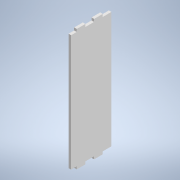
# Autodesk Inventor part: motorkap
Saved by Autodesk Inventor 2021 (Build 250183000, 183)
## iProperties
Created: 2022-02-02
Part Number: motorkap
Material: Generic
Document SubType Name: Modeling
Designer: ryan
Density: 1 g/cm^3
Appearance: Default
Author: ryan
Autodesk Inventor part; units mm, degrees
ref_plane "YZ Plane" through (0, 0, 0) normal (1, 0, 0) x (0, 1, 0)
ref_plane "XZ Plane" through (0, 0, 0) normal (0, 1, 0) x (-1, 0, 0)
ref_plane "XY Plane" through (0, 0, 0) normal (0, 0, 1) x (1, 0, 0)
sketch "Sketch1" plane through (0, 0, 0) normal (0, 1, 0) x (-1, 0, 0)
  line L0 (0, 0) -> (0, -10)
  line L1 (0, -10) -> (3, -10)
  line L2 (0, 0) -> (0, 10)
  line L3 (0, 10) -> (0, 20)
  line L4 (0, 20) -> (0, 30)
  line L5 (0, 30) -> (0, 36.5)
  line L6 (0, 36.5) -> (3, 36.5)
  line L7 (3, 36.5) -> (3, -10)
  line L8 (3, 30) -> (0, 30)
  line L9 (0, 20) -> (3, 20)
  line L10 (0, 10) -> (3, 10)
  line L11 (0, 0) -> (3, 0)
  dimension "d0" = 10
  dimension "d1" = 3
  dimension "d2" = 10
  dimension "d3" = 10
  dimension "d4" = 10
  dimension "d5" = 6.5
  dimension "d6" = 3
  constraints: 24 end point, 6 perpendicular, 6 point on line, 3 vertical
  measures "d0" distance of L0.start L0.end
  measures "d1" distance of L0.end L1.end
  measures "d2" distance of L0.start L2.end
  measures "d3" distance of L2.end L3.end
  measures "d4" distance of L3.end L4.end
  measures "d5" distance of L4.end L5.end
  measures "d6" distance of L5.end L6.end
extrude "Extrusion1" add sketch "Sketch1" along normal blind 3 contours L2 L10 L7 L11 | L4 L8 L7 L9
sketch "Sketch2" plane through (0, 3, 0) normal (0, 1, 0) x (1, 0, 0)
  line L0 (0, 0) -> (0, 10)
  line L1 (-3, -20) -> (-3, -30) projected
  line L2 (0, 10) -> (-3, 10)
  line L3 (-3, 10) -> (-3, -30)
  line L4 (-3, -30) -> (0, -30)
  line L5 (0, -30) -> (0, 10)
  line L6 (0, -30) -> (0, -36.5)
  line L7 (0, -36.5) -> (-3, -36.5)
  line L8 (-3, -36.5) -> (-3, -30)
  line L9 (-3, -30) -> (0, -30)
  line L10 (0, -30) -> (0, -36.5)
  dimension "d9" = 10
  dimension "d10" = 6.5
  constraints: 20 end point, 4 parallel, 2 horizontal, 2 perpendicular, 2 vertical
  measures "d9" distance of L0.start L0.end
  measures "d10" distance of L4.end L6.end
extrude "Extrusion2" add sketch "Sketch2" along normal blind 67
mirror "Mirror1" about plane through (-1.5, 70, 13.25) normal (0, 1, 0) of "Extrusion2", "Extrusion1"
body "Solid1"
